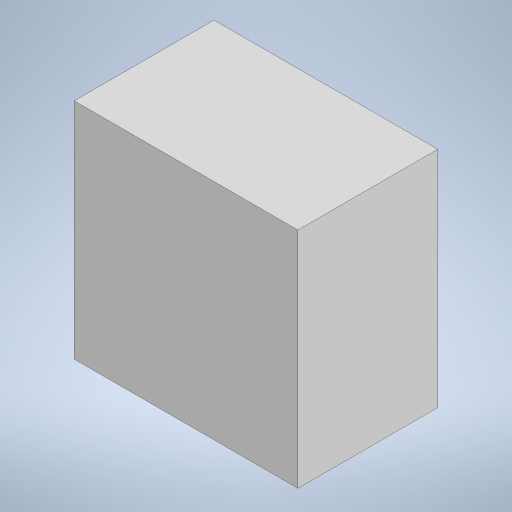
# Autodesk Inventor part: Box
Saved by Autodesk Inventor 2024 (Build 280153000, 153)
## iProperties
Created: 2026-05-30
Part Number: Box
Material: Generisch
Document SubType Name: Modeling
Designer: maxim
Density: 1 g/cm^3
Appearance: Vorgabe
Author: maxim
Autodesk Inventor part; units mm, degrees
ref_plane "YZ Plane" through (0, 0, 0) normal (1, 0, 0) x (0, 1, 0)
ref_plane "XZ Plane" through (0, 0, 0) normal (0, 1, 0) x (-1, 0, 0)
ref_plane "XY Plane" through (0, 0, 0) normal (0, 0, 1) x (1, 0, 0)
sketch "Skizze1" plane through (0, 0, 0) normal (0, 1, 0) x (-1, 0, 0)
  line L0 (-72, 72) -> (72, 72)
  line L1 (72, 72) -> (72, -72)
  line L2 (72, -72) -> (-72, -72)
  line L3 (-72, -72) -> (-72, 72)
  line L4 (-72, 72) -> (72, -72) construction
  line L5 (72, 72) -> (-72, -72) construction
  point P0 (0, 0)
  dimension "d0" = 144
  dimension "d1" = 144
  constraints: 12 end point, 2 midpoint, 2 parallel, 1 horizontal, 1 perpendicular
  measures "d0" distance of L1.end L2.end
  measures "d1" distance of L0.end L1.end
extrude "Extrusion1" add sketch "Skizze1" along normal blind 90
sketch "Skizze2" plane through (0, 90, 0) normal (0, 1, 0) x (1, 0, 0)
  line L0 (69, -69) -> (-69, -69)
  line L1 (-69, -69) -> (-69, 69)
  line L2 (-69, 69) -> (69, 69)
  line L3 (69, 69) -> (69, -69)
  line L4 (69, -69) -> (-69, 69) construction
  line L5 (-69, -69) -> (69, 69) construction
  line L6 (-72, 72) -> (-72, -72) projected
  line L7 (-72, -72) -> (72, -72) projected
  point P0 (0, 0)
  dimension "WALL" = 3
  dimension "d5" = 3
  constraints: 12 end point, 2 midpoint, 2 parallel, 1 horizontal, 1 perpendicular
  measures "WALL" distance between parallel lines of L6 L1
  measures "d5" distance between parallel lines of L7 L0
extrude "Extrusion2" cut sketch "Skizze2" against normal blind 87
sketch "Skizze7" plane through (-72, 0, -72) normal (-1, 0, 0) x (0, 0, 1)
  line L0 (89, 40) -> (139, 40)
  line L1 (139, 40) -> (139, 10)
  line L2 (139, 10) -> (89, 10)
  line L3 (89, 10) -> (89, 40)
  circle A0 centre (114, 45) radius 2.2
  line L4 (89, 25) -> (139, 25)
  circle A1 centre (114, 5) radius 2.2
  line L5 (144, 0) -> (144, 90) projected
  line L6 (0, 0) -> (144, 0) projected
  point P0 (72, 0)
  point P1 (114, 40)
  dimension "d35" = 30
  dimension "d36" = 50
  dimension "d37" = 4.4
  dimension "d38" = 40
  dimension "d41" = 5
  dimension "d42" = 10
  constraints: 10 end point, 3 midpoint, 2 centre point, 2 parallel, 1 horizontal, 1 perpendicular, 1 symmetric about line, 1 vertical alignment, 1 other
  measures "d35" distance of L0.end L1.end
  measures "d36" distance of L0.start L0.end
  measures "d37" diameter of A0
  measures "d38" diameter of A0.centre L4
  measures "d41" distance between parallel lines of L5 L1
  measures "d42" distance between parallel lines of L6 L2
extrude "Extrusion4" cut sketch "Skizze7" against normal blind 3
sketch "Skizze8" plane through (0, 90, 0) normal (0, 1, 0) x (1, 0, 0)
  line L0 (72, 72) -> (-72, 72) projected
  line L1 (72, 72) -> (56, 72)
  line L2 (56, 72) -> (56, 56)
  line L3 (56, 56) -> (72, 56)
  line L4 (72, 56) -> (72, 72)
  line L5 (-72, -72) -> (72, -72) projected
  line L6 (72, -72) -> (56, -72)
  line L7 (56, -72) -> (56, -56)
  line L8 (56, -56) -> (72, -56)
  line L9 (72, -56) -> (72, -72)
  line L10 (-72, -72) -> (-56, -72)
  line L11 (-56, -72) -> (-56, -56)
  line L12 (-56, -56) -> (-72, -56)
  line L13 (-72, -56) -> (-72, -72)
  line L14 (-72, 72) -> (-56, 72)
  line L15 (-56, 72) -> (-56, 56)
  line L16 (-56, 56) -> (-72, 56)
  line L17 (-72, 56) -> (-72, 72)
  line L18 (16, 72) -> (-16, 72)
  line L19 (-16, 72) -> (-16, 56)
  line L20 (-16, 56) -> (16, 56)
  line L21 (16, 56) -> (16, 72)
  line L22 (16, -72) -> (-16, -72)
  line L23 (-16, -72) -> (-16, -56)
  line L24 (-16, -56) -> (16, -56)
  line L25 (16, -56) -> (16, -72)
  line L26 (72, -72) -> (72, 72) projected
  line L27 (72, 16) -> (56, 16)
  line L28 (56, 16) -> (56, -16)
  line L29 (56, -16) -> (72, -16)
  line L30 (72, -16) -> (72, 16)
  line L31 (-72, 72) -> (-72, -72) projected
  line L32 (-72, 16) -> (-56, 16)
  line L33 (-56, 16) -> (-56, -16)
  line L34 (-56, -16) -> (-72, -16)
  line L35 (-72, -16) -> (-72, 16)
  point P0 (0, 0)
  point P1 (0, 56)
  point P2 (-56, 0)
  point P3 (56, 0)
  point P4 (-16, 72)
  point P5 (-72, -16)
  point P6 (-16, -72)
  dimension "d43" = 16
  dimension "INSERT_BLOCK" = 16
  dimension "d45" = 16
  dimension "d46" = 16
  dimension "d47" = 16
  dimension "d48" = 16
  dimension "d49" = 16
  dimension "d50" = 16
  dimension "d51" = 32
  dimension "d52" = 16
  dimension "d53" = 16
  dimension "d54" = 32
  dimension "d55" = 32
  dimension "d56" = 16
  constraints: 64 end point, 16 parallel, 8 horizontal, 8 perpendicular, 7 point on line, 3 midpoint, 2 horizontal alignment, 1 vertical alignment
  measures "d43" distance of L3.end L2.end
  measures "INSERT_BLOCK" distance of L2.end L1.end
  measures "d45" distance of L7.end L8.end
  measures "d46" distance of L6.end L7.end
  measures "d47" distance of L12.end L11.end
  measures "d48" distance of L11.end L10.end
  measures "d49" distance of L15.end L16.end
  measures "d50" distance of L14.end L15.end
  measures "d51" distance of L20.end L19.end
  measures "d52" distance of L19.end L18.end
  measures "d53" distance of L29.end L28.end
  measures "d54" distance of L28.end L27.end
  measures "d55" distance of L32.end L33.end
  measures "d56" distance of L33.end L34.end
extrude "Extrusion5" add sketch "Skizze8" against normal blind 12 contours L4 L3 L2 L0 | L21 L20 L19 L0 | L26 L29 L28 L27 | L15 L16 L17 L0 | L9 L5 L7 L8 | L32 L33 L34 L31 | L5 L23 L24 L25 | L12 L11 L5 L13
chamfer "Fasen1" distance 13 angle 45 8 edges at (69, 78, -62.5) (69, 78, 0) (69, 78, 62.5) (0, 78, 69) (-69, 78, 62.5) (-69, 78, 0) (0, 78, -69) (-69, 78, -62.5)
sketch "Skizze9" plane through (0, 90, 0) normal (0, 1, 0) x (1, 0, 0)
  circle A0 centre (64, 64) radius 2.2
  line L0 (72, 72) -> (-72, 72) projected
  line L1 (72, -72) -> (72, 72) projected
  circle A1 centre (64, 8) radius 2.2
  circle A2 centre (8, 64) radius 2.2
  circle A3 centre (8, 8) radius 2.2
  circle A4 centre (64, -8) radius 2.2
  circle A5 centre (64, -64) radius 2.2
  circle A6 centre (8, -64) radius 2.2
  circle A7 centre (8, -8) radius 2.2
  circle A8 centre (-8, 64) radius 2.2
  circle A9 centre (-8, 8) radius 2.2
  circle A10 centre (-64, 8) radius 2.2
  circle A11 centre (-64, 64) radius 2.2
  circle A12 centre (-8, -8) radius 2.2
  circle A13 centre (-8, -64) radius 2.2
  circle A14 centre (-64, -64) radius 2.2
  circle A15 centre (-64, -8) radius 2.2
  point P0 (0, 0)
  dimension "INSERT_DIAMETER" = 4.4
  dimension "d63" = 8
  dimension "d64" = 8
  dimension "d68" = 56
  dimension "d71" = 56
  dimension "d76" = 72
  dimension "d79" = 72
  constraints: 16 centre point, 2 horizontal, 2 vertical, 30 other
  measures "INSERT_DIAMETER" diameter of A0
  measures "d63" distance from line of L0 A0.centre
  measures "d64" distance from line of L1 A0.centre
  measures "d68" distance of A0.centre A1.centre
  measures "d71" distance of A0.centre A2.centre
  measures "d76" distance of A0.centre A4.centre
  measures "d79" distance of A0.centre A8.centre
extrude "Extrusion6" cut sketch "Skizze9" against normal blind 6
chamfer "Fasen2" distance 4 angle 45 12 edges at (56, 84, -56) (56, 84, -16) (56, 84, 16) (56, 84, 56) (16, 84, 56) (-16, 84, 56) (16, 84, -56) (-16, 84, -56) (-56, 84, -56) (-56, 84, -16) (-56, 84, 16) (-56, 84, 56)
sketch "Skizze10" plane through (-69, 3, 41.0835) normal (1, 0, 0) x (0, 0, -1)
  line L0 (3.0835, -3) -> (3.0835, 7)
  line L1 (3.0835, 7) -> (-4.9165, 7)
  line L2 (-4.9165, 7) -> (-4.9165, -3)
  line L3 (-4.9165, -3) -> (3.0835, -3)
  line L4 (3.0835, -3) -> (-4.9165, 7) construction
  line L5 (3.0835, 7) -> (-4.9165, -3) construction
  line L6 (3.0835, 47) -> (3.0835, 37)
  line L7 (3.0835, 37) -> (-4.9165, 37)
  line L8 (-4.9165, 37) -> (-4.9165, 47)
  line L9 (-4.9165, 47) -> (3.0835, 47)
  line L10 (3.0835, 47) -> (-4.9165, 37) construction
  line L11 (3.0835, 37) -> (-4.9165, 47) construction
  point P0 (41.0835, -3)
  point P1 (-0.9165, 2)
  point P2 (-0.9165, 42)
  dimension "d93" = 8
  dimension "d94" = 8
  constraints: 24 end point, 4 midpoint, 4 parallel, 2 perpendicular
  measures "d93" distance of L1.end L0.end
  measures "d94" distance of L6.end L7.end
extrude "Extrusion7" add sketch "Skizze10" along normal blind 4
sketch "Skizze11" plane through (0, 3, 0) normal (0, 1, 0) x (1, 0, 0)
  circle A0 centre (-57, 59) radius 4
  circle A1 centre (35.5, -11) radius 4
  line L0 (-69, 69) -> (69, 69) projected
  line L1 (-69, -38) -> (-69, 69) projected
  point P0 (0, 0)
  dimension "d95" = 8
  dimension "d96" = 8
  dimension "d97" = 10
  dimension "d98" = 12
  dimension "d99" = 70
  dimension "d100" = 92.5
  constraints: 2 centre point
  measures "d95" diameter of A0
  measures "d96" diameter of A1
  measures "d97" distance from line of L0 A0.centre
  measures "d98" distance from line of L1 A0.centre
  measures "d99" vertical distance of A1.centre A0.centre
  measures "d100" horizontal distance of A1.centre A0.centre
extrude "Extrusion8" add sketch "Skizze11" along normal blind 2
sketch "Skizze12" plane through (35.5, 5, 11) normal (0, 1, 0) x (1, 0, 0)
  circle A0 centre (0, 0) radius 2.2
  circle A1 centre (-92.5, 70) radius 4 projected
  circle A2 centre (-92.5, 70) radius 2.2
  point P0 (-35.5, 11)
  dimension "d103" = 4.4
  dimension "d104" = 4.4
  constraints: 2 centre point, 1 coincident
  measures "d103" diameter of A0
  measures "d104" diameter of A2
extrude "Extrusion9" cut sketch "Skizze12" against normal blind 4 contours A0 | A2
sketch "Skizze13" plane through (72, 0, -72) normal (0, 0, -1) x (-1, 0, 0)
  circle A0 centre (26.5, 80) radius 4
  line L0 (0, 90) -> (144, 90) projected
  line L1 (0, 0) -> (0, 90) projected
  circle A1 centre (117.5, 80) radius 4
  circle A2 centre (26.5, 9) radius 4
  circle A3 centre (117.5, 9) radius 4
  point P0 (72, 0)
  point P1 (72, 90)
  dimension "d107" = 8
  dimension "d108" = 45.5
  dimension "d109" = 10
  dimension "d112" = 91
  dimension "d115" = 71
  constraints: 4 centre point, 1 horizontal, 1 midpoint, 1 vertical, 6 other
  measures "d107" diameter of A0
  measures "d108" horizontal distance of point (72, 90) A0.centre
  measures "d109" distance from line of A0.centre L0
  measures "d112" distance of A0.centre A1.centre
  measures "d115" distance of A0.centre A2.centre
extrude "Extrusion10" add sketch "Skizze13" along normal blind 2
sketch "Skizze14" plane through (45.5, 80, -74) normal (0, 0, -1) x (-1, 0, 0)
  circle A0 centre (0, 0) radius 4 projected
  circle A1 centre (0, 0) radius 2.2
  circle A2 centre (91, 0) radius 4 projected
  circle A3 centre (91, 0) radius 2.2
  circle A4 centre (0, -71) radius 4 projected
  circle A5 centre (0, -71) radius 2.2
  circle A6 centre (91, -71) radius 4 projected
  circle A7 centre (91, -71) radius 2.2
  point P0 (45.5, -80)
  dimension "d120" = 4.4
  dimension "d121" = 4.4
  dimension "d122" = 4.4
  dimension "d123" = 4.4
  constraints: 4 centre point, 4 coincident
  measures "d120" diameter of A1
  measures "d121" diameter of A3
  measures "d122" diameter of A5
  measures "d123" diameter of A7
extrude "Extrusion11" cut sketch "Skizze14" against normal up to surface (5 mm away) contours A1 | A3 | A5 | A7
chamfer "Fasen3" distance 2 angle 45 4 edges at (49.5, 80, -72) (-41.5, 80, -72) (-41.5, 9, -72) (49.5, 9, -72)
sketch "Skizze15" plane through (72, 0, -72) normal (0, 0, -1) x (-1, 0, 0)
  line L0 (24.5, 30) -> (24.5, 60) construction
  line L1 (29.5, 30) -> (29.5, 60)
  line L2 (19.5, 60) -> (19.5, 30)
  arc A0 (19.5, 30) -> (29.5, 30) centre (24.5, 30) ccw
  arc A1 (29.5, 60) -> (19.5, 60) centre (24.5, 60) ccw
  circle A2 centre (29.5, 30) radius 5
  circle A3 centre (19.5, 30) radius 5
  circle A4 centre (26.5, 80) radius 2.2 projected
  line L3 (0, 0) -> (0, 90) projected
  point P0 (72, 0)
  point P1 (24.5, 45)
  point P2 (24.5, 65)
  point P3 (19.5, 45)
  point P4 (0, 45)
  point P5 (29.5, 35)
  point P6 (19.5, 35)
  point P7 (22, 25.6699)
  point P8 (27, 25.6699)
  dimension "d129" = 30
  dimension "d130" = 10
  dimension "d136" = 2
  constraints: 8 end point, 5 point on circle, 5 tangent, 3 centre point, 3 midpoint, 2 coincident, 1 horizontal alignment, 1 parallel, 1 vertical, 3 other
  measures "d129" distance of L0.end L0.start
  measures "d130" distance of L2.end L1.start
  measures "d136" horizontal distance of A4.centre point (24.5, 65)
extrude "Extrusion12" cut sketch "Skizze15" against normal up to surface (3 mm away) contours A0 A2 L1 | L1 A2 A0 | A2 A3 L2 A1 L1 | A0 A3 A2 | A3 A0 L2 | A3 L2 A0
pattern_linear "Rechteckige Anordnung1" count 2 spacing 95 along (-1, 0, 0) of "Extrusion12"
sketch "Skizze16" plane through (72, 0, -72) normal (0, 0, -1) x (-1, 0, 0)
  circle A0 centre (8.5, 80) radius 2.5
  circle A1 centre (26.5, 80) radius 2.2 projected
  circle A2 centre (117.5, 80) radius 2.2 projected
  line L0 (0, 90) -> (144, 90) projected
  line L1 (0, 0) -> (0, 90) projected
  circle A3 centre (135.5, 80) radius 2.5
  circle A4 centre (8.5, 9) radius 2.5
  circle A5 centre (135.5, 9) radius 2.5
  point P0 (72, 0)
  dimension "d137" = 5
  dimension "d138" = 18
  dimension "d141" = 127
  dimension "d144" = 71
  constraints: 4 centre point, 1 horizontal, 1 horizontal alignment, 1 vertical, 6 other
  measures "d137" diameter of A0
  measures "d138" distance of A0.centre A1.centre
  measures "d141" distance of A0.centre A3.centre
  measures "d144" distance of A0.centre A4.centre
extrude "Extrusion13" cut sketch "Skizze16" against normal blind 3 contours A0 | A3 | A4 | A5
sketch "Skizze18" plane through (-69, 3, -69) normal (0, 0, 1) x (1, 0, 0)
  line L0 (0, 62) -> (0, 0) projected
  line L1 (0, 0) -> (11, 0)
  line L2 (11, 0) -> (11, 11)
  line L3 (11, 11) -> (0, 11)
  line L4 (0, 11) -> (0, 0)
  line L5 (138, 62) -> (138, 0) projected
  line L6 (138, 0) -> (127, 0)
  line L7 (127, 0) -> (127, 11)
  line L8 (127, 11) -> (138, 11)
  line L9 (138, 11) -> (138, 0)
  point P0 (69, -3)
  dimension "d151" = 11
  dimension "d152" = 11
  dimension "d153" = 11
  dimension "d154" = 11
  constraints: 16 end point, 4 parallel, 2 horizontal, 2 perpendicular
  measures "d151" distance of L2.end L1.end
  measures "d152" distance of L7.end L8.end
  measures "d153" distance of L6.end L7.end
  measures "d154" distance of L2.end L3.end
extrude "Extrusion15" add sketch "Skizze18" along normal blind 1.5
sketch "Skizze19" plane through (0, 3, 0) normal (0, 1, 0) x (1, 0, 0)
  line L0 (69, -69) -> (-69, -69) projected
  line L1 (69, 67.5) -> (69, -69) projected
  circle A0 centre (54, 37) radius 4
  circle A1 centre (54, -54) radius 4
  circle A2 centre (-2, -54) radius 4
  point P0 (0, 0)
  dimension "d157" = 91
  dimension "d158" = 56
  dimension "d159" = 15
  dimension "d160" = 15
  dimension "d161" = 8
  dimension "d162" = 8
  dimension "d163" = 8
  constraints: 3 centre point, 3 coincident, 1 horizontal alignment, 1 vertical alignment
  measures "d157" distance of point (54, -54) point (54, 37)
  measures "d158" distance of point (-2, -54) point (54, -54)
  measures "d159" distance from line of L0 point (54, -54)
  measures "d160" distance from line of L1 point (54, -54)
  measures "d161" diameter of A0
  measures "d162" diameter of A1
  measures "d163" diameter of A2
extrude "Extrusion16" add sketch "Skizze19" along normal blind 35
sketch "Skizze20" plane through (54, 38, -37) normal (0, 1, 0) x (1, 0, 0)
  circle A0 centre (0, 0) radius 4 projected
  circle A1 centre (0, 0) radius 2.2
  circle A2 centre (0, -91) radius 4 projected
  circle A3 centre (0, -91) radius 2.2
  circle A4 centre (-56, -91) radius 4 projected
  circle A5 centre (-56, -91) radius 2.2
  point P0 (-54, -37)
  dimension "d166" = 4.4
  dimension "d167" = 4.4
  dimension "d168" = 4.4
  constraints: 3 centre point, 3 coincident
  measures "d166" diameter of A1
  measures "d167" diameter of A3
  measures "d168" diameter of A5
extrude "Extrusion17" cut sketch "Skizze20" against normal blind 6 contours A1 | A3 | A5
equation "\"d5\" = WALL"
equation "\"d6\" = BOX_HEIGHT - WALL"
equation "\"d39\" = WALL"
equation "\"BOX_HEIGHT\" = 90"
